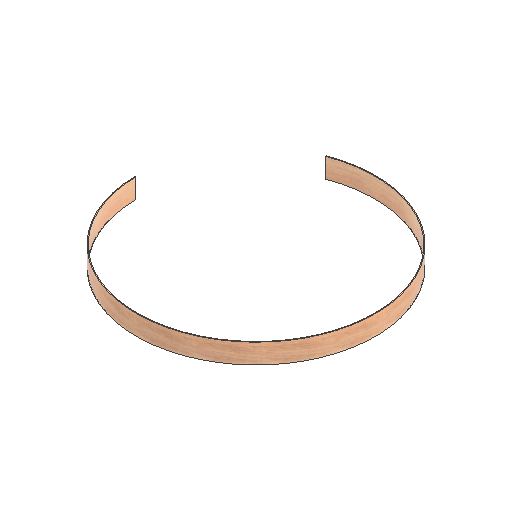
# Autodesk Inventor part: Edge Band - Platform A Outer
Saved by Autodesk Inventor 2021 (Build 250183000, 183)
## iProperties
Created: 2020-05-12
Part Number: Edge Band - Platform A Outer
Material: Wood (Birch)
Document SubType Name: Modeling
Designer: Dan Wikman
Density: 0.55 g/cm^3
Appearance: Birch - Natural Polished
Mass: 669.676 g
Surface Area: 6339.48 cm^2
Volume: 1217.59 cm^3
Author: Dan Wikman
Autodesk Inventor part; units mm, degrees
ref_plane "YZ Plane" through (0, 0, 0) normal (1, 0, 0) x (0, 1, 0)
ref_plane "XZ Plane" through (0, 0, 0) normal (0, 1, 0) x (-1, 0, 0)
ref_plane "XY Plane" through (0, 0, 0) normal (0, 0, 1) x (1, 0, 0)
sketch "Sketch1" plane through (0, 0, 0) normal (0, 1, 0) x (-1, 0, 0)
  circle A0 centre (0, 0) radius 600
  circle A1 centre (0, 0) radius 604
  dimension "d0" = 1200
  dimension "d1" = 1208
  constraints: 2 centre point, 2 coincident
  measures "d0" diameter of A0
  measures "d1" diameter of A1
extrude "Extrusion1" add sketch "Sketch1" along normal blind 100
sketch "Sketch2" plane through (0, 0, 0) normal (0, -1, 0) x (1, 0, 0)
  line L0 (-737.5363, 12.1167) -> (-600.0118, 8.1785) projected
  line L1 (-256.3877, -691.6444) -> (-210.1448, -562.0678) projected
  circle A0 centre (0, 0) radius 600 projected
  line L2 (-210.1221, -562.0042) -> (-211.4667, -565.7719)
  circle A1 centre (0, 0) radius 604 projected
  line L3 (-599.9441, 8.1765) -> (-603.943, 8.2911)
  point P0 (-599.9443, 8.1765)
  point P1 (-603.9431, 8.2911)
  constraints: 4 end point, 3 point on line, 4 other
extrude "Extrusion2" cut sketch "Sketch2" against normal blind 100 contours L0 L3 A0 L2 L1 A1 picked at (-484.3692, -358.2492)
body "Solid1"
